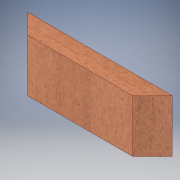
# Autodesk Inventor part: dou_long
Saved by Autodesk Inventor 2019 (Build 230136000, 136)
## iProperties
Created: 2019-11-15
Part Number: dou_long
Material: Красное дерево
Document SubType Name: Modeling
Designer: stepa
Density: 0.512 g/cm^3
Appearance: Красное дерево — натуральный — полированный
Mass: 106.218 g
Surface Area: 396.549 cm^2
Volume: 207.457 cm^3
Author: stepa
Autodesk Inventor part; units mm, degrees
ref_plane "YZ Plane" through (0, 0, 0) normal (1, 0, 0) x (0, 1, 0)
ref_plane "XZ Plane" through (0, 0, 0) normal (0, 1, 0) x (-1, 0, 0)
ref_plane "XY Plane" through (0, 0, 0) normal (0, 0, 1) x (1, 0, 0)
sketch "Эскиз1" plane through (0, 0, 0) normal (0, 1, 0) x (-1, 0, 0)
  line L0 (0, 0) -> (-220, 0)
  line L1 (-220, 0) -> (-220, -30)
  line L2 (-220, -30) -> (0, -30)
  line L3 (0, -30) -> (0, 0)
  dimension "d0" = 220
  dimension "d1" = 30
  constraints: 8 end point, 2 parallel, 1 horizontal, 1 perpendicular
  measures "d0" distance of L2.end L1.end
  measures "d1" distance of L1.end L0.end
extrude "Выдавливание1" add sketch "Эскиз1" along normal blind 80
chamfer "Фаска1" distance 30 angle 45 2 edges at (0, 40, 0) (220, 40, 0)
